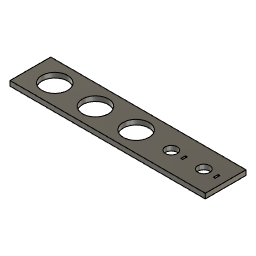
led-lamp-button-test (Autodesk Fusion 360 design; units mm, degrees)
Autodesk Fusion 360 part; units mm, degrees
sketch "Sketch1" plane through (0, 0, 0) normal (0, 0, 1) x (1, 0, 0)
  line L0 (0, 0) -> (120, 0)
  line L1 (120, 0) -> (120, 25)
  line L2 (120, 25) -> (0, 25)
  line L3 (0, 25) -> (0, 0)
  circle A0 centre (15, 12.5) radius 7.95
  circle A1 centre (40, 12.5) radius 7.95
  circle A2 centre (65, 12.5) radius 7.95
  circle A3 centre (86.6, 12.5) radius 3.65
  circle A4 centre (106.6, 12.5) radius 3.65
  line L4 (93.9, 13.9) -> (95, 13.9)
  line L5 (95, 13.9) -> (95, 11.1)
  line L6 (95, 11.1) -> (93.9, 11.1)
  line L7 (93.9, 11.1) -> (93.9, 13.9)
  line L8 (113.9, 13.9) -> (115, 13.9)
  line L9 (115, 13.9) -> (115, 11.1)
  line L10 (115, 11.1) -> (113.9, 11.1)
  line L11 (113.9, 11.1) -> (113.9, 13.9)
  line L12 (86.6, 12.5) -> (93.9, 12.5)
  line L13 (106.6, 12.5) -> (113.9, 12.5)
  line L14 (15, 12.5) -> (40, 12.5)
  line L15 (40, 12.5) -> (65, 12.5)
  line L16 (15, 12.5) -> (0, 12.5)
  dimension "d1" = 15.9
  dimension "d2" = 7.3
  dimension "d3" = 20
  dimension "d4" = 7.3
  dimension "d5" = 1.1
  dimension "d6" = 2.8
  dimension "d7" = 7.3
  dimension "d8" = 2.8
  dimension "d9" = 1.1
  dimension "d10" = 25
  dimension "d11" = 15
  dimension "d12" = 25
  dimension "d13" = 120
  dimension "d14" = 5
  constraint horizontal L0
  constraint vertical L1
  constraint horizontal L2
  constraint vertical L3
  constraint coincident L0.start L3.end
  constraint equal A0 A1
  constraint equal A1 A2
  constraint equal A3 A4
  constraint horizontal L4
  constraint vertical L5
  constraint horizontal L6
  constraint vertical L7
  constraint horizontal L8
  constraint vertical L9
  constraint horizontal L10
  constraint vertical L11
  constraint coincident A3.centre L12.start
  constraint midpoint L7 L12.end
  constraint horizontal L12
  constraint coincident A4.centre L13.start
  constraint midpoint L11 L13.end
  constraint horizontal L13
  constraint collinear L12 L13
  constraint coincident A0.centre L14.start
  constraint coincident A1.centre L14.end
  constraint parallel L2 L14
  constraint coincident A2.centre L15.end
  constraint parallel L2 L15
  constraint equal L14 L15
  constraint collinear L12 L15
  constraint midpoint L3 L16.end
  constraint horizontal L16
  measures "d1" diameter of A0
  measures "d2" diameter of A3
  measures "d3" distance of A3.centre A4.centre
  measures "d4" distance of A3.centre L7
  measures "d5" distance of L5 L7
  measures "d6" distance of L4.end L5.end
  measures "d7" distance of A4.centre L13.end
  measures "d8" distance of L8.end L9.end
  measures "d9" distance of L8.start L8.end
  measures "d10" distance of A0.centre A1.centre
  measures "d11" distance of L3 A0.centre
  measures "d12" distance of L0.start L2.end
  measures "d13" distance of L1.end L2.end
  measures "d14" distance of L1 L9
extrude "Extrude1" add sketch "Sketch1" along normal blind 3
